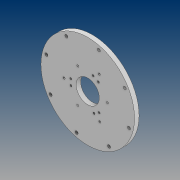
# Autodesk Inventor part: foreas_2_2_old
Saved by Autodesk Inventor 2021 (Build 250183000, 183)
## iProperties
Created: 2021-01-08
Part Number: foreas_2_2_old
Material: Generic
Document SubType Name: Modeling
Designer: Angelos
Density: 1 g/cm^3
Appearance: Default
Author: Angelos
Autodesk Inventor part; units mm, degrees
(part 1 of 3)
ref_plane "YZ Plane" through (0, 0, 0) normal (1, 0, 0) x (0, 1, 0)
ref_plane "XZ Plane" through (0, 0, 0) normal (0, 1, 0) x (-1, 0, 0)
ref_plane "XY Plane" through (0, 0, 0) normal (0, 0, 1) x (1, 0, 0)
sketch "Sketch2" plane through (0, 0, 0) normal (0, 0, 1) x (1, 0, 0)
  circle A0 centre (0, 0) radius 235
  circle A1 centre (115.1116, 204.8763) radius 10
  circle A2 centre (53.4628, 161.3745) radius 10
  circle A3 centre (0, 0) radius 170
  circle A4 centre (105.4319, 133.3571) radius 10
  circle A5 centre (115.1116, 204.8763) radius 10
  line L0 (114.1116, 214.8763) -> (115.1116, 213.4482)
  line L1 (115.1116, 213.4482) -> (116.1116, 214.8763)
  circle A6 centre (-234.9839, -2.7486) radius 10
  circle A7 centre (-166.4858, -34.3871) radius 10
  circle A8 centre (-168.2066, 24.6282) radius 10
  circle A9 centre (119.8723, -202.1278) radius 10
  circle A10 centre (113.023, -126.9874) radius 10
  circle A11 centre (62.7746, -157.9853) radius 10
  line L2 (107.6882, 200.5904) -> (105.9514, 200.7423)
  line L3 (106.9514, 199.0103) -> (107.6882, 200.5904)
  line L4 (122.5351, 200.5904) -> (123.2719, 199.0103)
  line L5 (124.2719, 200.7423) -> (122.5351, 200.5904)
  line L6 (-242.4074, -7.0345) -> (-244.1442, -6.8825)
  line L7 (-243.1442, -8.6146) -> (-242.4074, -7.0345)
  line L8 (-225.8237, -6.8825) -> (-227.5605, -7.0345)
  line L9 (-227.5605, -7.0345) -> (-226.8237, -8.6146)
  line L10 (-235.9839, 7.2514) -> (-234.9839, 5.8233)
  line L11 (-234.9839, 5.8233) -> (-233.9839, 7.2514)
  line L12 (127.2957, -206.4137) -> (128.0325, -207.9938)
  line L13 (129.0325, -206.2617) -> (127.2957, -206.4137)
  line L14 (118.8723, -192.1278) -> (119.8723, -193.5559)
  line L15 (119.8723, -193.5559) -> (120.8723, -192.1278)
  line L16 (111.712, -207.9938) -> (112.4488, -206.4137)
  line L17 (112.4488, -206.4137) -> (110.712, -206.2617)
  circle A12 centre (0, 0) radius 465
  circle A13 centre (0, 0) radius 196
  line L18 (0, 0) -> (105.4319, 133.3571)
  line L19 (119.8723, -202.1278) -> (0, 0)
  circle A14 centre (196, 0) radius 10
  line L20 (0, 0) -> (196, 0)
  circle A15 centre (-98, 169.741) radius 10
  circle A16 centre (-98, -169.741) radius 10
  point P0 (155.1924, 176.4662)
  point P1 (155.1924, 176.4662)
  point P2 (155.1924, 176.4662)
  point P3 (128.9755, -206.2667)
  point P4 (128.0083, -207.9419)
  point P5 (111.7362, -207.9419)
  point P6 (110.769, -206.2667)
  point P7 (118.9051, -192.1747)
  point P8 (120.8395, -192.1747)
  point P9 (123.2477, 199.0622)
  point P10 (106.9756, 199.0622)
  point P11 (106.0084, 200.7374)
  point P12 (114.1445, 214.8294)
  point P13 (116.0788, 214.8294)
  point P14 (124.2149, 200.7374)
  point P15 (-234.0168, 7.2046)
  point P16 (-225.8807, -6.8875)
  point P17 (-226.8479, -8.5627)
  point P18 (-243.12, -8.5627)
  point P19 (-244.0872, -6.8875)
  point P20 (-235.9511, 7.2046)
  dimension "d44" = 470
  dimension "d45" = 20
  dimension "d46" = 20
  dimension "d47" = 170
  dimension "d48" = 20
  dimension "d49" = 20
  dimension "d50" = 20
  dimension "d51" = 360
  dimension "d52" = 234.9839
  dimension "d55" = 360
  dimension "d59" = 360
  dimension "d61" = 930
  dimension "d76" = 392
  dimension "d84" = 20
  dimension "d94" = 360
  constraints: 42 end point, 16 centre point, 6 coincident, 2 point on circle, 91 other
  measures "d45" diameter of A1
  measures "d46" diameter of A2
  measures "d47" distance of A2.centre point (0, 0)
  measures "d48" diameter of A4
  measures "d50" diameter of A5
  measures "d52" horizontal distance of point (0, 0) A6.centre
  measures "d61" diameter of A12
  measures "d76" diameter of A13
  measures "d84" diameter of A14
extrude "Extrusion2" add sketch "Sketch2" along normal blind 20 contours A0 A9 A6 A1 | A1 L4 A0 | A0 L4 L5 A1 | L15 L14 A9 | A1 L2 L3 | L17 L16 A9 A0 | A0 A9 L17 | A9 L12 L13 | A6 L11 A0 | A0 L11 L10 A6 | A1 L1 L0 | L6 L7 A6 | L9 L8 A6 | A2 A3 A8 A7 A11 L19 A13 A16 A15 A14 L20 A4 | A2 A3 A4 L18 L19 A11 A7 A8 | A4 A3 L20 L18 | L20 A3 A10 L19 | L20 A14 A13 L19 A3 A10 | L20 A13 A14 | A14 A13 L20 | A14 A13 | A16 A13 | A13 A16 | A15 A13 | A13 A15 | A12
thread "Thread1" size "M20x2.5" class "6H" standard "ANSI Metric M Profile" full length
thread "Thread2" size "M20x2.5" class "6H" standard "ANSI Metric M Profile" full length
thread "Thread3" size "M20x2.5" class "6H" standard "ANSI Metric M Profile" full length
thread "Thread4" size "M20x2.5" class "6H" standard "ANSI Metric M Profile" full length
thread "Thread5" size "M20x2.5" class "6H" standard "ANSI Metric M Profile" full length
thread "Thread6" size "M20x2.5" class "6H" standard "ANSI Metric M Profile" full length
extrude "Extrusion3" cut sketch "Sketch2" along normal through all contours L20 A13 A14 | A14 A13 L20 | A14 A13 | A16 A13 | A13 A16 | A15 A13 | A13 A15
sketch "Sketch3" plane through (0, 0, 20) normal (0, 0, 1) x (1, 0, 0)
  circle A0 centre (0, 0) radius 115
  dimension "d96" = 230
  constraints: 1 centre point, 1 coincident
  measures "d96" diameter of A0
extrude "Extrusion4" cut sketch "Sketch3" against normal through all
sketch "Sketch4" plane through (0, 0, 20) normal (0, 0, 1) x (1, 0, 0)
  circle A0 centre (0, 0) radius 425
  circle A1 centre (110.6339, 410.3476) radius 15
  line L0 (0, 425) -> (110.6339, 410.3476)
  dimension "d103" = 360
  dimension "d99" = 850
  dimension "d112" = 111.6
  dimension "d113" = 0
  dimension "d114" = 0
  constraints: 3 point on circle, 2 centre point, 2 end point, 1 coincident, 1 other
  measures "d99" diameter of A0
  measures "d112" distance of L0.start L0.end
  measures "d113" distance of L0.end A1.centre
  measures "d114" horizontal distance of point (0, 0) L0.start
extrude "Extrusion5" cut sketch "Sketch4" against normal blind 50 contours A1 A0 | A0 L0 A1 | L0 A0 A1 picked at (104.0654, 411.4285) picked at (112.4556, 404.9089)
pattern_circular "Circular Pattern1" count 8 over 360 about axis through (0, 0, -10) along (0, 0, 1) of "Extrusion5"
sketch "Sketch6" plane through (0, 0, 0) normal (0, 0, -1) x (-1, 0, 0)
  circle A0 centre (0, 0) radius 465
  circle A1 centre (0, 0) radius 115
  dimension "d123" = 930
  constraints: 2 centre point, 2 coincident
  measures "d123" diameter of A0
extrude "Extrusion7" add sketch "Sketch6" along normal blind 25
sketch "Sketch7" plane through (0, 0, -25) normal (0, 0, -1) x (-1, 0, 0)
  circle A0 centre (0, 0) radius 130
  circle A1 centre (0, 130) radius 8
  circle A2 centre (-123.6373, 40.1722) radius 8
  circle A3 centre (-76.4121, -105.1722) radius 8
  circle A4 centre (76.4121, -105.1722) radius 8
  circle A5 centre (123.6373, 40.1722) radius 8
  dimension "d126" = 260
  dimension "d127" = 16
  dimension "d184" = 360
  constraints: 5 centre point, 1 coincident, 1 vertical alignment, 13 other
  measures "d127" diameter of A1
extrude "Extrusion8" cut sketch "Sketch7" against normal blind 15 contours A5 A0 | A0 A5 | A4 A0 | A0 A4 | A1 A0 | A0 A1 | A3 A0 | A0 A3 | A2 A0 | A0 A2
sketch "Sketch8" plane through (0, 0, 0) normal (1, 0, 0) x (0, 1, 0)
  line L0 (138, -10) -> (122, -10) projected
  line L1 (138, -10) -> (122, -10)
  line L2 (122, -10) -> (130, -2)
  line L3 (138, -10) -> (130, -2)
  line L4 (138, -10) -> (157.9972, -10) construction
  line L5 (138, -10) -> (130.4376, -10)
  line L6 (130, -2) -> (130, -10)
  line L7 (130, -2) -> (138, -2) construction
  point P0 (0, 0)
  dimension "d176" = 45
  dimension "d177" = 135
  dimension "d178" = 90
  constraints: 14 end point, 2 collinear, 2 horizontal, 1 midpoint, 1 perpendicular, 1 point on line
  measures "d176" angle of L1 L2
  measures "d177" angle of L4 L3
  measures "d178" angle of L6 L7
revolve "Revolution1" cut sketch "Sketch8" angle 360 about axis through (0, 130, -2) along (0, 0, -1) contours L0 L6 L3
pattern_circular "Circular Pattern3" count 5 over 360 about axis through (0, 0, 20) along (0, 0, -1) of "Revolution1"
sketch "Sketch9" plane through (0, 0, 20) normal (0, 0, 1) x (1, 0, 0)
  circle A0 centre (-166.4858, -34.3871) radius 10 projected
  circle A1 centre (-166.4858, -34.3871) radius 10
  circle A2 centre (-168.2066, 24.6282) radius 10 projected
  circle A3 centre (-168.2066, 24.6282) radius 10
  point P0 (0, 0)
  constraints: 2 centre point, 2 coincident
extrude "Extrusion9" cut sketch "Sketch9" against normal through all
pattern_circular "Circular Pattern4" count 3 over 360 about axis through (0, 0, 20) along (0, 0, -1) of "Extrusion9"
sketch "Sketch10" plane through (0, 0, 20) normal (0, 0, 1) x (1, 0, 0)
  circle A0 centre (-368.3896, -211.9296) radius 15 projected
  circle A1 centre (-368.3896, -211.9296) radius 15
  point P0 (0, 0)
  constraints: 1 centre point, 1 coincident
extrude "Extrusion10" cut sketch "Sketch10" against normal through all
pattern_circular "Circular Pattern5" count 8 over 360 about axis through (0, 0, 20) along (0, 0, -1) of "Extrusion10"
thread "Thread7" size "M30x3.5" class "6H" standard "ANSI Metric M Profile" full length
thread "Thread8" size "M30x3.5" class "6H" standard "ANSI Metric M Profile" full length
thread "Thread9" size "M30x3.5" class "6H" standard "ANSI Metric M Profile" full length
thread "Thread10" size "M30x3.5" class "6H" standard "ANSI Metric M Profile" full length
thread "Thread11" size "M30x3.5" class "6H" standard "ANSI Metric M Profile" full length
thread "Thread12" size "M30x3.5" class "6H" standard "ANSI Metric M Profile" full length
thread "Thread13" size "M30x3.5" class "6H" standard "ANSI Metric M Profile" full length
thread "Thread14" size "M30x3.5" class "6H" standard "ANSI Metric M Profile" full length
thread "Thread15" size "M20x2.5" class "6H" standard "ANSI Metric M Profile" full length
thread "Thread16" size "M20x2.5" class "6H" standard "ANSI Metric M Profile" full length
thread "Thread17" size "M20x2.5" class "6H" standard "ANSI Metric M Profile" full length
thread "Thread18" size "M20x2.5" class "6H" standard "ANSI Metric M Profile" full length
thread "Thread19" size "M20x2.5" class "6H" standard "ANSI Metric M Profile" full length
thread "Thread20" size "M20x2.5" class "6H" standard "ANSI Metric M Profile" full length
pattern_circular "Circular Pattern6" count 5 over 360 about axis through (0, 0, -10) along (0, 0, 1) of "Revolution1"
thread "Thread21" size "M16x2" class "6H" standard "ANSI Metric M Profile" full length
thread "Thread22" size "M16x2" class "6H" standard "ANSI Metric M Profile" full length
thread "Thread23" size "M16x2" class "6H" standard "ANSI Metric M Profile" full length
thread "Thread24" size "M16x2" class "6H" standard "ANSI Metric M Profile" full length
thread "Thread25" size "M16x2" class "6H" standard "ANSI Metric M Profile" full length
sketch "Sketch11" plane through (0, 0, -25) normal (0, 0, -1) x (-1, 0, 0)
  circle A0 centre (0, 0) radius 115 projected
  circle A1 centre (0, 0) radius 318.114
  circle A2 centre (0, 0) radius 359.1006
  spline S0 degree 2 poles (-321.1231, 5.4547) (-320.2877, 5.4473) (-318.9493, 4.758) (-318.5787, 4.1862) knots 0 0 0 1 2 2 2
  spline S1 degree 2 poles (-318.5787, 4.1862) (-318.2912, 3.719) (-318.102, 2.7632) (-318.1087, 2.0217) knots 0 0 0 1 2 2 2
  line L0 (-318.1087, 2.0217) -> (-318.1212, 0.6179)
  line L1 (-318.1212, 0.6179) -> (-324.221, 0.6724)
  line L2 (-324.221, 0.6724) -> (-324.2085, 2.0614)
  spline S2 degree 2 poles (-324.2085, 2.0614) (-324.2008, 2.9215) (-323.9351, 3.898) (-323.7046, 4.2419) knots 0 0 0 1 2 2 2
  spline S3 degree 2 poles (-323.7046, 4.2419) (-323.3088, 4.8267) (-322.0129, 5.4627) (-321.1231, 5.4547) knots 0 0 0 1 2 2 2
  spline S4 degree 2 poles (-321.1406, 4.6096) (-321.8425, 4.6158) (-322.8402, 4.1601) (-323.1261, 3.7029) knots 0 0 0 1 2 2 2
  spline S5 degree 2 poles (-323.1261, 3.7029) (-323.3218, 3.3784) (-323.5014, 2.6434) (-323.5063, 2.0947) knots 0 0 0 1 2 2 2
  line L3 (-323.5063, 2.0947) -> (-323.5118, 1.4768)
  line L4 (-323.5118, 1.4768) -> (-318.8159, 1.4348)
  line L5 (-318.8159, 1.4348) -> (-318.8103, 2.0527)
  spline S6 degree 2 poles (-318.8103, 2.0527) (-318.8055, 2.5915) (-318.9712, 3.4087) (-319.2006, 3.7419) knots 0 0 0 1 2 2 2
  spline S7 degree 2 poles (-319.2006, 3.7419) (-319.4835, 4.1696) (-320.4288, 4.6032) (-321.1406, 4.6096) knots 0 0 0 1 2 2 2
  line L6 (-318.0044, 8.4321) -> (-318.0583, 6.0699)
  line L7 (-318.0583, 6.0699) -> (-318.681, 6.0841)
  line L8 (-318.681, 6.0841) -> (-318.6633, 6.8599)
  line L9 (-318.6633, 6.8599) -> (-323.5163, 6.9706)
  line L10 (-323.5163, 6.9706) -> (-323.534, 6.1947)
  line L11 (-323.534, 6.1947) -> (-324.1567, 6.2089)
  line L12 (-324.1567, 6.2089) -> (-324.1028, 8.5712)
  line L13 (-324.1028, 8.5712) -> (-323.4801, 8.557)
  line L14 (-323.4801, 8.557) -> (-323.4978, 7.7811)
  line L15 (-323.4978, 7.7811) -> (-318.6448, 7.6704)
  line L16 (-318.6448, 7.6704) -> (-318.6271, 8.4463)
  line L17 (-318.6271, 8.4463) -> (-318.0044, 8.4321)
  spline S8 degree 2 poles (-323.2222, 13.948) (-322.8043, 14.2788) (-321.6044, 14.6202) (-320.8437, 14.592) knots 0 0 0 1 2 2 2
  spline S9 degree 2 poles (-320.8437, 14.592) (-320.1027, 14.5645) (-318.9162, 14.1446) (-318.5243, 13.7739) knots 0 0 0 1 2 2 2
  spline S10 degree 2 poles (-318.5243, 13.7739) (-318.1134, 13.3827) (-317.7452, 12.3748) (-317.7673, 11.777) knots 0 0 0 1 2 2 2
  spline S11 degree 2 poles (-317.7673, 11.777) (-317.7902, 11.1596) (-318.2467, 10.1871) (-318.6701, 9.8417) knots 0 0 0 1 2 2 2
  spline S12 degree 2 poles (-318.6701, 9.8417) (-319.0882, 9.506) (-320.2926, 9.1747) (-321.0435, 9.2026) knots 0 0 0 1 2 2 2
  spline S13 degree 2 poles (-321.0435, 9.2026) (-321.8091, 9.2309) (-322.9609, 9.6545) (-323.3677, 10.0208) knots 0 0 0 1 2 2 2
  spline S14 degree 2 poles (-323.3677, 10.0208) (-323.7596, 10.3915) (-324.1427, 11.4) (-324.12, 12.0125) knots 0 0 0 1 2 2 2
  spline S15 degree 2 poles (-324.12, 12.0125) (-324.0969, 12.635) (-323.6252, 13.6167) (-323.2222, 13.948) knots 0 0 0 1 2 2 2
  spline S16 degree 2 poles (-320.875, 13.7472) (-321.4777, 13.7696) (-322.421, 13.5424) (-322.7361, 13.3166) knots 0 0 0 1 2 2 2
  spline S17 degree 2 poles (-322.7361, 13.3166) (-323.0612, 13.0863) (-323.4026, 12.4163) (-323.4184, 11.9915) knots 0 0 0 1 2 2 2
  spline S18 degree 2 poles (-323.4184, 11.9915) (-323.4347, 11.5518) (-323.1529, 10.8785) (-322.8362, 10.6145) knots 0 0 0 1 2 2 2
  spline S19 degree 2 poles (-322.8362, 10.6145) (-322.534, 10.3609) (-321.6049, 10.0693) (-321.0122, 10.0473) knots 0 0 0 1 2 2 2
  spline S20 degree 2 poles (-321.0122, 10.0473) (-319.8118, 10.0028) (-318.4999, 10.9633) (-318.4686, 11.808) knots 0 0 0 1 2 2 2
  spline S21 degree 2 poles (-318.4686, 11.808) (-318.4373, 12.6527) (-319.6746, 13.7027) (-320.875, 13.7472) knots 0 0 0 1 2 2 2
  spline S22 degree 2 poles (-317.4907, 17.9128) (-317.5264, 17.2662) (-317.9804, 16.217) (-318.4015, 15.8541) knots 0 0 0 1 2 2 2
  spline S23 degree 2 poles (-318.4015, 15.8541) (-318.8275, 15.4915) (-320.0446, 15.1478) (-320.8195, 15.1906) knots 0 0 0 1 2 2 2
  spline S24 degree 2 poles (-320.8195, 15.1906) (-321.5549, 15.2312) (-322.6968, 15.7102) (-323.0902, 16.118) knots 0 0 0 1 2 2 2
  spline S25 degree 2 poles (-323.0902, 16.118) (-323.4695, 16.5103) (-323.8439, 17.6202) (-323.8082, 18.2668) knots 0 0 0 1 2 2 2
  spline S26 degree 2 poles (-323.8082, 18.2668) (-323.791, 18.5777) (-323.6711, 19.1355) (-323.5779, 19.3878) knots 0 0 0 1 2 2 2
  spline S27 degree 2 poles (-323.5779, 19.3878) (-323.5072, 19.5918) (-323.2622, 20.0833) (-323.1748, 20.2319) knots 0 0 0 1 2 2 2
  line L18 (-323.1748, 20.2319) -> (-322.1975, 20.1779)
  line L19 (-322.1975, 20.1779) -> (-322.2014, 20.1088)
  spline S28 degree 2 poles (-322.2014, 20.1088) (-322.3431, 19.9632) (-322.6026, 19.6557) (-322.7572, 19.3672) knots 0 0 0 1 2 2 2
  spline S29 degree 2 poles (-322.7572, 19.3672) (-322.8942, 19.1272) (-323.0923, 18.4995) (-323.1125, 18.1343) knots 0 0 0 1 2 2 2
  spline S30 degree 2 poles (-323.1125, 18.1343) (-323.161, 17.2557) (-321.8982, 16.0968) (-320.7975, 16.036) knots 0 0 0 1 2 2 2
  spline S31 degree 2 poles (-320.7975, 16.036) (-320.1855, 16.0021) (-319.2516, 16.2377) (-318.9207, 16.4917) knots 0 0 0 1 2 2 2
  spline S32 degree 2 poles (-318.9207, 16.4917) (-318.5904, 16.7359) (-318.2188, 17.458) (-318.1932, 17.9219) knots 0 0 0 1 2 2 2
  spline S33 degree 2 poles (-318.1932, 17.9219) (-318.1744, 18.2625) (-318.2355, 18.9491) (-318.3214, 19.1865) knots 0 0 0 1 2 2 2
  line L20 (-318.3214, 19.1865) -> (-319.8959, 19.2735)
  line L21 (-319.8959, 19.2735) -> (-319.9738, 17.8619)
  line L22 (-319.9738, 17.8619) -> (-320.6846, 17.9011)
  line L23 (-320.6846, 17.9011) -> (-320.5624, 20.1123)
  line L24 (-320.5624, 20.1123) -> (-317.9021, 19.9654)
  spline S34 degree 2 poles (-317.9021, 19.9654) (-317.8414, 19.8085) (-317.6581, 19.2736) (-317.6062, 19.048) knots 0 0 0 1 2 2 2
  spline S35 degree 2 poles (-317.6062, 19.048) (-317.534, 18.742) (-317.4719, 18.2534) (-317.4907, 17.9128) knots 0 0 0 1 2 2 2
  line L25 (-317.4276, 20.9589) -> (-323.512, 21.394)
  line L26 (-323.512, 21.394) -> (-323.2398, 25.2005)
  line L27 (-323.2398, 25.2005) -> (-322.52, 25.149)
  line L28 (-322.52, 25.149) -> (-322.7343, 22.1512)
  line L29 (-322.7343, 22.1512) -> (-321.0678, 22.032)
  line L30 (-321.0678, 22.032) -> (-320.8678, 24.8277)
  line L31 (-320.8678, 24.8277) -> (-320.148, 24.7762)
  line L32 (-320.148, 24.7762) -> (-320.3479, 21.9805)
  line L33 (-320.3479, 21.9805) -> (-318.0896, 21.819)
  line L34 (-318.0896, 21.819) -> (-317.8753, 24.8169)
  line L35 (-317.8753, 24.8169) -> (-317.1554, 24.7654)
  line L36 (-317.1554, 24.7654) -> (-317.4276, 20.9589)
  line L37 (-316.7037, 30.0006) -> (-316.7833, 29.0945)
  line L38 (-316.7833, 29.0945) -> (-322.2589, 26.8659)
  line L39 (-322.2589, 26.8659) -> (-317.0194, 26.4058)
  line L40 (-317.0194, 26.4058) -> (-317.0855, 25.6524)
  line L41 (-317.0855, 25.6524) -> (-323.1622, 26.186)
  line L42 (-323.1622, 26.186) -> (-323.0614, 27.3334)
  line L43 (-323.0614, 27.3334) -> (-318.0354, 29.3583)
  line L44 (-318.0354, 29.3583) -> (-322.8465, 29.7808)
  line L45 (-322.8465, 29.7808) -> (-322.7803, 30.5342)
  line L46 (-322.7803, 30.5342) -> (-316.7037, 30.0006)
  line L47 (-316.3638, 33.3448) -> (-316.6027, 30.994)
  line L48 (-316.6027, 30.994) -> (-317.2224, 31.057)
  line L49 (-317.2224, 31.057) -> (-317.1439, 31.8291)
  line L50 (-317.1439, 31.8291) -> (-321.9733, 32.32)
  line L51 (-321.9733, 32.32) -> (-322.0518, 31.5479)
  line L52 (-322.0518, 31.5479) -> (-322.6715, 31.6109)
  line L53 (-322.6715, 31.6109) -> (-322.4325, 33.9617)
  line L54 (-322.4325, 33.9617) -> (-321.8128, 33.8987)
  line L55 (-321.8128, 33.8987) -> (-321.8913, 33.1266)
  line L56 (-321.8913, 33.1266) -> (-317.0619, 32.6356)
  line L57 (-317.0619, 32.6356) -> (-316.9834, 33.4078)
  line L58 (-316.9834, 33.4078) -> (-316.3638, 33.3448)
  spline S36 degree 2 poles (-315.9587, 36.02) (-316.0338, 35.3619) (-316.4141, 34.4699) (-316.6571, 34.0847) knots 0 0 0 1 2 2 2
  line L59 (-316.6571, 34.0847) -> (-317.6688, 34.2001)
  line L60 (-317.6688, 34.2001) -> (-317.6621, 34.259)
  spline S37 degree 2 poles (-317.6621, 34.259) (-317.2435, 34.6142) (-316.7161, 35.574) (-316.6629, 36.0406) knots 0 0 0 1 2 2 2
  spline S38 degree 2 poles (-316.6629, 36.0406) (-316.5867, 36.7086) (-317.0638, 37.4546) (-317.5206, 37.5067) knots 0 0 0 1 2 2 2
  spline S39 degree 2 poles (-317.5206, 37.5067) (-317.884, 37.5481) (-318.3767, 37.2411) (-318.534, 36.866) knots 0 0 0 1 2 2 2
  spline S40 degree 2 poles (-318.534, 36.866) (-318.6445, 36.595) (-318.8057, 36.1407) (-318.9339, 35.8021) knots 0 0 0 1 2 2 2
  spline S41 degree 2 poles (-318.9339, 35.8021) (-319.0533, 35.4973) (-319.3603, 35.0298) (-319.5835, 34.8612) knots 0 0 0 1 2 2 2
  spline S42 degree 2 poles (-319.5835, 34.8612) (-319.8062, 34.6976) (-320.37, 34.5529) (-320.7236, 34.5932) knots 0 0 0 1 2 2 2
  spline S43 degree 2 poles (-320.7236, 34.5932) (-321.4603, 34.6773) (-322.3263, 35.9403) (-322.2249, 36.8292) knots 0 0 0 1 2 2 2
  spline S44 degree 2 poles (-322.2249, 36.8292) (-322.1666, 37.34) (-321.8622, 38.2208) (-321.6264, 38.5869) knots 0 0 0 1 2 2 2
  line L61 (-321.6264, 38.5869) -> (-320.6637, 38.4771)
  line L62 (-320.6637, 38.4771) -> (-320.6705, 38.4182)
  spline S45 degree 2 poles (-320.6705, 38.4182) (-320.9687, 38.1587) (-321.4647, 37.2998) (-321.5213, 36.8037) knots 0 0 0 1 2 2 2
  spline S46 degree 2 poles (-321.5213, 36.8037) (-321.5851, 36.2438) (-321.1386, 35.4914) (-320.7113, 35.4426) knots 0 0 0 1 2 2 2
  spline S47 degree 2 poles (-320.7113, 35.4426) (-320.3282, 35.3989) (-319.825, 35.7545) (-319.6781, 36.1258) knots 0 0 0 1 2 2 2
  spline S48 degree 2 poles (-319.6781, 36.1258) (-319.5802, 36.3734) (-319.3188, 37.0948) (-319.2172, 37.332) knots 0 0 0 1 2 2 2
  spline S49 degree 2 poles (-319.2172, 37.332) (-318.9545, 37.9339) (-318.1173, 38.4255) (-317.5525, 38.3611) knots 0 0 0 1 2 2 2
  spline S50 degree 2 poles (-317.5525, 38.3611) (-317.1939, 38.3202) (-316.5394, 37.952) (-316.3284, 37.6642) knots 0 0 0 1 2 2 2
  spline S51 degree 2 poles (-316.3284, 37.6642) (-316.0962, 37.3442) (-315.8954, 36.575) (-315.9587, 36.02) knots 0 0 0 1 2 2 2
  line L63 (-315.1957, 42.9923) -> (-320.5237, 43.726)
  line L64 (-320.5237, 43.726) -> (-320.8029, 41.6987)
  line L65 (-320.8029, 41.6987) -> (-321.5179, 41.7971)
  line L66 (-321.5179, 41.7971) -> (-320.8489, 46.655)
  line L67 (-320.8489, 46.655) -> (-320.1339, 46.5565)
  line L68 (-320.1339, 46.5565) -> (-320.4131, 44.5292)
  line L69 (-320.4131, 44.5292) -> (-315.0851, 43.7954)
  line L70 (-315.0851, 43.7954) -> (-315.1957, 42.9923)
  spline S52 degree 2 poles (-314.3461, 48.1028) (-314.4463, 47.448) (-314.8606, 46.5713) (-315.1181, 46.1956) knots 0 0 0 1 2 2 2
  line L71 (-315.1181, 46.1956) -> (-316.1247, 46.3497)
  line L72 (-316.1247, 46.3497) -> (-316.1157, 46.4084)
  spline S53 degree 2 poles (-316.1157, 46.4084) (-315.6838, 46.7473) (-315.12, 47.6862) (-315.0489, 48.1504) knots 0 0 0 1 2 2 2
  spline S54 degree 2 poles (-315.0489, 48.1504) (-314.9472, 48.8149) (-315.3954, 49.5787) (-315.8498, 49.6482) knots 0 0 0 1 2 2 2
  spline S55 degree 2 poles (-315.8498, 49.6482) (-316.2114, 49.7036) (-316.7156, 49.4157) (-316.887, 49.0469) knots 0 0 0 1 2 2 2
  spline S56 degree 2 poles (-316.887, 49.0469) (-317.0079, 48.7803) (-317.1864, 48.3326) (-317.3275, 47.9991) knots 0 0 0 1 2 2 2
  spline S57 degree 2 poles (-317.3275, 47.9991) (-317.4584, 47.6991) (-317.7832, 47.2437) (-318.0127, 47.0838) knots 0 0 0 1 2 2 2
  spline S58 degree 2 poles (-318.0127, 47.0838) (-318.2414, 46.9288) (-318.8104, 46.8059) (-319.1622, 46.8597) knots 0 0 0 1 2 2 2
  spline S59 degree 2 poles (-319.1622, 46.8597) (-319.8951, 46.9719) (-320.712, 48.2672) (-320.5766, 49.1516) knots 0 0 0 1 2 2 2
  spline S60 degree 2 poles (-320.5766, 49.1516) (-320.4988, 49.6598) (-320.1609, 50.5282) (-319.9112, 50.8851) knots 0 0 0 1 2 2 2
  line L73 (-319.9112, 50.8851) -> (-318.9535, 50.7384)
  line L74 (-318.9535, 50.7384) -> (-318.9625, 50.6798)
  spline S61 degree 2 poles (-318.9625, 50.6798) (-319.2705, 50.4319) (-319.799, 49.5927) (-319.8745, 49.0991) knots 0 0 0 1 2 2 2
  spline S62 degree 2 poles (-319.8745, 49.0991) (-319.9598, 48.5421) (-319.5424, 47.7731) (-319.1173, 47.708) knots 0 0 0 1 2 2 2
  spline S63 degree 2 poles (-319.1173, 47.708) (-318.7362, 47.6497) (-318.2197, 47.9857) (-318.0587, 48.3511) knots 0 0 0 1 2 2 2
  spline S64 degree 2 poles (-318.0587, 48.3511) (-317.9514, 48.5947) (-317.6626, 49.3056) (-317.5519, 49.5387) knots 0 0 0 1 2 2 2
  spline S65 degree 2 poles (-317.5519, 49.5387) (-317.2663, 50.1301) (-316.4109, 50.5893) (-315.849, 50.5032) knots 0 0 0 1 2 2 2
  spline S66 degree 2 poles (-315.849, 50.5032) (-315.4922, 50.4486) (-314.8523, 50.0556) (-314.6525, 49.76) knots 0 0 0 1 2 2 2
  spline S67 degree 2 poles (-314.6525, 49.76) (-314.4328, 49.4313) (-314.2616, 48.655) (-314.3461, 48.1028) knots 0 0 0 1 2 2 2
  line L75 (-313.6445, 53.1511) -> (-314.0307, 50.8199)
  line L76 (-314.0307, 50.8199) -> (-314.6451, 50.9217)
  line L77 (-314.6451, 50.9217) -> (-314.5183, 51.6874)
  line L78 (-314.5183, 51.6874) -> (-319.3073, 52.4807)
  line L79 (-319.3073, 52.4807) -> (-319.4342, 51.715)
  line L80 (-319.4342, 51.715) -> (-320.0487, 51.8168)
  line L81 (-320.0487, 51.8168) -> (-319.6625, 54.148)
  line L82 (-319.6625, 54.148) -> (-319.048, 54.0462)
  line L83 (-319.048, 54.0462) -> (-319.1749, 53.2805)
  line L84 (-319.1749, 53.2805) -> (-314.3858, 52.4872)
  line L85 (-314.3858, 52.4872) -> (-314.259, 53.2528)
  line L86 (-314.259, 53.2528) -> (-313.6445, 53.1511)
  spline S68 degree 2 poles (-312.9522, 56.467) (-313.0566, 55.8831) (-313.6274, 54.9658) (-314.086, 54.6762) knots 0 0 0 1 2 2 2
  spline S69 degree 2 poles (-314.086, 54.6762) (-314.5397, 54.3857) (-315.778, 54.2005) (-316.5371, 54.3363) knots 0 0 0 1 2 2 2
  spline S70 degree 2 poles (-316.5371, 54.3363) (-317.2914, 54.4712) (-318.3418, 55.0558) (-318.6901, 55.4947) knots 0 0 0 1 2 2 2
  spline S71 degree 2 poles (-318.6901, 55.4947) (-319.0296, 55.927) (-319.2771, 56.9857) (-319.1684, 57.594) knots 0 0 0 1 2 2 2
  spline S72 degree 2 poles (-319.1684, 57.594) (-319.1144, 57.8957) (-318.9319, 58.4104) (-318.8238, 58.622) knots 0 0 0 1 2 2 2
  spline S73 degree 2 poles (-318.8238, 58.622) (-318.7257, 58.8054) (-318.4734, 59.1771) (-318.3307, 59.3574) knots 0 0 0 1 2 2 2
  line L87 (-318.3307, 59.3574) -> (-317.3672, 59.1851)
  line L88 (-317.3672, 59.1851) -> (-317.3785, 59.1218)
  spline S74 degree 2 poles (-317.3785, 59.1218) (-317.495, 59.0322) (-317.8267, 58.75) (-318.0007, 58.5351) knots 0 0 0 1 2 2 2
  spline S75 degree 2 poles (-318.0007, 58.5351) (-318.1681, 58.329) (-318.4253, 57.8176) (-318.488, 57.4672) knots 0 0 0 1 2 2 2
  spline S76 degree 2 poles (-318.488, 57.4672) (-318.5567, 57.0828) (-318.3632, 56.3401) (-318.1076, 56.0283) knots 0 0 0 1 2 2 2
  spline S77 degree 2 poles (-318.1076, 56.0283) (-317.8463, 55.7204) (-316.9674, 55.2719) (-316.3883, 55.1684) knots 0 0 0 1 2 2 2
  spline S78 degree 2 poles (-316.3883, 55.1684) (-315.7703, 55.0578) (-314.8267, 55.1954) (-314.4741, 55.3984) knots 0 0 0 1 2 2 2
  spline S79 degree 2 poles (-314.4741, 55.3984) (-314.132, 55.5984) (-313.7093, 56.2208) (-313.6414, 56.6003) knots 0 0 0 1 2 2 2
  spline S80 degree 2 poles (-313.6414, 56.6003) (-313.5796, 56.9458) (-313.6446, 57.5651) (-313.7302, 57.8164) knots 0 0 0 1 2 2 2
  spline S81 degree 2 poles (-313.7302, 57.8164) (-313.8176, 58.058) (-314.022, 58.4311) (-314.0979, 58.54) knots 0 0 0 1 2 2 2
  line L89 (-314.0979, 58.54) -> (-314.0875, 58.5984)
  line L90 (-314.0875, 58.5984) -> (-313.1337, 58.4278)
  spline S82 degree 2 poles (-313.1337, 58.4278) (-313.077, 58.2118) (-312.9693, 57.831) (-312.9359, 57.5689) knots 0 0 0 1 2 2 2
  spline S83 degree 2 poles (-312.9359, 57.5689) (-312.8953, 57.2904) (-312.8877, 56.8271) (-312.9522, 56.467) knots 0 0 0 1 2 2 2
  line L91 (-311.7311, 63.444) -> (-311.8873, 62.6485)
  line L92 (-311.8873, 62.6485) -> (-314.8171, 63.2236)
  line L93 (-314.8171, 63.2236) -> (-315.3579, 60.4684)
  line L94 (-315.3579, 60.4684) -> (-312.428, 59.8933)
  line L95 (-312.428, 59.8933) -> (-312.5842, 59.0978)
  line L96 (-312.5842, 59.0978) -> (-318.57, 60.2727)
  line L97 (-318.57, 60.2727) -> (-318.4138, 61.0682)
  line L98 (-318.4138, 61.0682) -> (-316.0661, 60.6074)
  line L99 (-316.0661, 60.6074) -> (-315.5253, 63.3626)
  line L100 (-315.5253, 63.3626) -> (-317.873, 63.8234)
  line L101 (-317.873, 63.8234) -> (-317.7169, 64.6189)
  line L102 (-317.7169, 64.6189) -> (-311.7311, 63.444)
  line L103 (-310.7438, 68.111) -> (-311.4781, 64.6536)
  line L104 (-311.4781, 64.6536) -> (-317.445, 65.921)
  line L105 (-317.445, 65.921) -> (-317.2765, 66.714)
  line L106 (-317.2765, 66.714) -> (-312.0156, 65.5966)
  line L107 (-312.0156, 65.5966) -> (-311.4497, 68.2609)
  line L108 (-311.4497, 68.2609) -> (-310.7438, 68.111)
  line L109 (-310.7518, 68.0925) -> (-316.243, 71.4518)
  line L110 (-316.243, 71.4518) -> (-316.0213, 72.4254)
  line L111 (-316.0213, 72.4254) -> (-309.617, 73.0763)
  line L112 (-309.617, 73.0763) -> (-309.8069, 72.2424)
  line L113 (-309.8069, 72.2424) -> (-311.5927, 72.0812)
  line L114 (-311.5927, 72.0812) -> (-312.1096, 69.811)
  line L115 (-312.1096, 69.811) -> (-310.5696, 68.8926)
  line L116 (-310.5696, 68.8926) -> (-310.7518, 68.0925)
  line L117 (-312.3169, 72.018) -> (-315.3268, 71.735)
  line L118 (-315.3268, 71.735) -> (-312.735, 70.1816)
  line L119 (-312.735, 70.1816) -> (-312.3169, 72.018)
  line L120 (-308.4049, 78.0367) -> (-308.6548, 77.0139)
  line L121 (-308.6548, 77.0139) -> (-311.9403, 75.5217)
  line L122 (-311.9403, 75.5217) -> (-311.6359, 75.0809)
  line L123 (-311.6359, 75.0809) -> (-309.2685, 74.5025)
  line L124 (-309.2685, 74.5025) -> (-309.4609, 73.7149)
  line L125 (-309.4609, 73.7149) -> (-315.3866, 75.1629)
  line L126 (-315.3866, 75.1629) -> (-315.1941, 75.9504)
  line L127 (-315.1941, 75.9504) -> (-312.4714, 75.2851)
  line L128 (-312.4714, 75.2851) -> (-314.6004, 78.3802)
  line L129 (-314.6004, 78.3802) -> (-314.3657, 79.3406)
  line L130 (-314.3657, 79.3406) -> (-312.3194, 76.2403)
  line L131 (-312.3194, 76.2403) -> (-308.4049, 78.0367)
  line L132 (-307.746, 80.5623) -> (-308.336, 78.2742)
  line L133 (-308.336, 78.2742) -> (-308.9391, 78.4297)
  line L134 (-308.9391, 78.4297) -> (-308.7453, 79.1813)
  line L135 (-308.7453, 79.1813) -> (-313.4459, 80.3932)
  line L136 (-313.4459, 80.3932) -> (-313.6397, 79.6417)
  line L137 (-313.6397, 79.6417) -> (-314.2428, 79.7972)
  line L138 (-314.2428, 79.7972) -> (-313.6529, 82.0852)
  line L139 (-313.6529, 82.0852) -> (-313.0498, 81.9297)
  line L140 (-313.0498, 81.9297) -> (-313.2435, 81.1782)
  line L141 (-313.2435, 81.1782) -> (-308.5429, 79.9663)
  line L142 (-308.5429, 79.9663) -> (-308.3492, 80.7178)
  line L143 (-308.3492, 80.7178) -> (-307.746, 80.5623)
  spline S84 degree 2 poles (-306.9431, 83.1461) (-307.1163, 82.5068) (-307.6265, 81.6822) (-307.9247, 81.3379) knots 0 0 0 1 2 2 2
  line L144 (-307.9247, 81.3379) -> (-308.9076, 81.6042)
  line L145 (-308.9076, 81.6042) -> (-308.8921, 81.6615)
  spline S85 degree 2 poles (-308.8921, 81.6615) (-308.4247, 81.9497) (-307.7589, 82.8192) (-307.6361, 83.2725) knots 0 0 0 1 2 2 2
  spline S86 degree 2 poles (-307.6361, 83.2725) (-307.4603, 83.9214) (-307.8198, 84.7306) (-308.2635, 84.8509) knots 0 0 0 1 2 2 2
  spline S87 degree 2 poles (-308.2635, 84.8509) (-308.6166, 84.9465) (-309.1499, 84.7172) (-309.3618, 84.37) knots 0 0 0 1 2 2 2
  spline S88 degree 2 poles (-309.3618, 84.37) (-309.5118, 84.1187) (-309.7396, 83.6938) (-309.9172, 83.3784) knots 0 0 0 1 2 2 2
  spline S89 degree 2 poles (-309.9172, 83.3784) (-310.0811, 83.095) (-310.455, 82.679) (-310.701, 82.5459) knots 0 0 0 1 2 2 2
  spline S90 degree 2 poles (-310.701, 82.5459) (-310.9458, 82.4176) (-311.5249, 82.3594) (-311.8684, 82.4525) knots 0 0 0 1 2 2 2
  spline S91 degree 2 poles (-311.8684, 82.4525) (-312.5841, 82.6464) (-313.2502, 84.0253) (-313.0162, 84.8889) knots 0 0 0 1 2 2 2
  spline S92 degree 2 poles (-313.0162, 84.8889) (-312.8817, 85.3851) (-312.4483, 86.21) (-312.1601, 86.5365) knots 0 0 0 1 2 2 2
  line L146 (-312.1601, 86.5365) -> (-311.2249, 86.2832)
  line L147 (-311.2249, 86.2832) -> (-311.2404, 86.2259)
  spline S93 degree 2 poles (-311.2404, 86.2259) (-311.5743, 86.0142) (-312.1939, 85.2397) (-312.3244, 84.7578) knots 0 0 0 1 2 2 2
  spline S94 degree 2 poles (-312.3244, 84.7578) (-312.4718, 84.2139) (-312.1436, 83.4028) (-311.7285, 83.2904) knots 0 0 0 1 2 2 2
  spline S95 degree 2 poles (-311.7285, 83.2904) (-311.3563, 83.1895) (-310.8053, 83.4653) (-310.6043, 83.8103) knots 0 0 0 1 2 2 2
  spline S96 degree 2 poles (-310.6043, 83.8103) (-310.4702, 84.0403) (-310.1033, 84.7143) (-309.9671, 84.9334) knots 0 0 0 1 2 2 2
  spline S97 degree 2 poles (-309.9671, 84.9334) (-309.6168, 85.489) (-308.7152, 85.849) (-308.1665, 85.7004) knots 0 0 0 1 2 2 2
  spline S98 degree 2 poles (-308.1665, 85.7004) (-307.8182, 85.606) (-307.2265, 85.1435) (-307.0612, 84.8273) knots 0 0 0 1 2 2 2
  spline S99 degree 2 poles (-307.0612, 84.8273) (-306.8798, 84.476) (-306.797, 83.6853) (-306.9431, 83.1461) knots 0 0 0 1 2 2 2
  spline S100 degree 2 poles (-306.3956, 92.6511) (-305.9453, 92.518) (-305.2703, 91.9938) (-305.0886, 91.6669) knots 0 0 0 1 2 2 2
  spline S101 degree 2 poles (-305.0886, 91.6669) (-304.8954, 91.3263) (-304.8091, 90.5894) (-304.9253, 90.196) knots 0 0 0 1 2 2 2
  spline S102 degree 2 poles (-304.9253, 90.196) (-305.0416, 89.8025) (-305.499, 89.2315) (-305.8374, 89.0634) knots 0 0 0 1 2 2 2
  spline S103 degree 2 poles (-305.8374, 89.0634) (-306.2447, 88.8539) (-307.4122, 88.8278) (-308.1896, 89.0576) knots 0 0 0 1 2 2 2
  spline S104 degree 2 poles (-308.1896, 89.0576) (-308.9528, 89.2832) (-310.0882, 89.9589) (-310.4466, 90.4205) knots 0 0 0 1 2 2 2
  spline S105 degree 2 poles (-310.4466, 90.4205) (-310.7983, 90.8698) (-310.9991, 92.0219) (-310.8043, 92.6809) knots 0 0 0 1 2 2 2
  spline S106 degree 2 poles (-310.8043, 92.6809) (-310.7469, 92.8752) (-310.6081, 93.2054) (-310.5276, 93.3207) knots 0 0 0 1 2 2 2
  line L148 (-310.5276, 93.3207) -> (-309.7739, 93.098)
  line L149 (-309.7739, 93.098) -> (-309.7837, 93.0648)
  spline S107 degree 2 poles (-309.7837, 93.0648) (-309.8728, 92.9726) (-310.09, 92.6038) (-310.1573, 92.3762) knots 0 0 0 1 2 2 2
  spline S108 degree 2 poles (-310.1573, 92.3762) (-310.373, 91.6462) (-309.6518, 90.4588) (-308.7099, 90.0877) knots 0 0 0 1 2 2 2
  spline S109 degree 2 poles (-308.7099, 90.0877) (-308.8216, 90.4248) (-308.8612, 91.0757) (-308.7575, 91.4265) knots 0 0 0 1 2 2 2
  spline S110 degree 2 poles (-308.7575, 91.4265) (-308.6567, 91.7678) (-308.3679, 92.2392) (-308.0766, 92.4572) knots 0 0 0 1 2 2 2
  spline S111 degree 2 poles (-308.0766, 92.4572) (-307.7396, 92.7081) (-306.8981, 92.7996) (-306.3956, 92.6511) knots 0 0 0 1 2 2 2
  spline S112 degree 2 poles (-306.5978, 91.8449) (-306.9581, 91.9514) (-307.5024, 91.9061) (-307.7347, 91.7479) knots 0 0 0 1 2 2 2
  spline S113 degree 2 poles (-307.7347, 91.7479) (-307.9042, 91.6279) (-308.0997, 91.263) (-308.1599, 91.0591) knots 0 0 0 1 2 2 2
  spline S114 degree 2 poles (-308.1599, 91.0591) (-308.2412, 90.7842) (-308.228, 90.2184) (-308.1458, 89.9209) knots 0 0 0 1 2 2 2
  spline S115 degree 2 poles (-308.1458, 89.9209) (-308.0619, 89.891) (-307.9035, 89.8339) (-307.7802, 89.7974) knots 0 0 0 1 2 2 2
  spline S116 degree 2 poles (-307.7802, 89.7974) (-307.1734, 89.6181) (-306.3591, 89.6352) (-306.1115, 89.7579) knots 0 0 0 1 2 2 2
  spline S117 degree 2 poles (-306.1115, 89.7579) (-305.8776, 89.8691) (-305.6242, 90.186) (-305.5639, 90.3898) knots 0 0 0 1 2 2 2
  spline S118 degree 2 poles (-305.5639, 90.3898) (-305.4238, 90.8639) (-305.9246, 91.6459) (-306.5978, 91.8449) knots 0 0 0 1 2 2 2
  line L150 (-303.1707, 96.3728) -> (-304.2887, 92.781)
  line L151 (-304.2887, 92.781) -> (-305.1147, 93.0381)
  spline S119 degree 2 poles (-305.1147, 93.0381) (-305.3577, 93.5382) (-305.8181, 94.4374) (-306.0787, 94.8809) knots 0 0 0 1 2 2 2
  spline S120 degree 2 poles (-306.0787, 94.8809) (-306.6032, 95.7741) (-307.3297, 96.5335) (-307.797, 96.679) knots 0 0 0 1 2 2 2
  spline S121 degree 2 poles (-307.797, 96.679) (-308.0425, 96.7554) (-308.4576, 96.7189) (-308.6182, 96.6188) knots 0 0 0 1 2 2 2
  spline S122 degree 2 poles (-308.6182, 96.6188) (-308.7788, 96.5186) (-309.0085, 96.1966) (-309.0761, 95.9795) knots 0 0 0 1 2 2 2
  spline S123 degree 2 poles (-309.0761, 95.9795) (-309.1407, 95.7719) (-309.1691, 95.3147) (-309.1491, 95.0962) knots 0 0 0 1 2 2 2
  spline S124 degree 2 poles (-309.1491, 95.0962) (-309.1344, 94.9105) (-309.0411, 94.5449) (-309.0044, 94.43) knots 0 0 0 1 2 2 2
  line L152 (-309.0044, 94.43) -> (-309.0176, 94.3875)
  line L153 (-309.0176, 94.3875) -> (-309.8483, 94.646)
  spline S125 degree 2 poles (-309.8483, 94.646) (-309.8914, 94.9235) (-309.8538, 95.8592) (-309.7334, 96.2463) knots 0 0 0 1 2 2 2
  spline S126 degree 2 poles (-309.7334, 96.2463) (-309.4792, 97.0628) (-308.329, 97.7143) (-307.5927, 97.4852) knots 0 0 0 1 2 2 2
  spline S127 degree 2 poles (-307.5927, 97.4852) (-307.2481, 97.3779) (-306.7223, 97.0382) (-306.5209, 96.8202) knots 0 0 0 1 2 2 2
  spline S128 degree 2 poles (-306.5209, 96.8202) (-306.3101, 96.5993) (-305.9376, 96.0329) (-305.7674, 95.7314) knots 0 0 0 1 2 2 2
  spline S129 degree 2 poles (-305.7674, 95.7314) (-305.4808, 95.2384) (-304.9024, 94.0695) (-304.7359, 93.7226) knots 0 0 0 1 2 2 2
  line L154 (-304.7359, 93.7226) -> (-303.8457, 96.5829)
  line L155 (-303.8457, 96.5829) -> (-303.1707, 96.3728)
  line L156 (-301.8479, 100.4338) -> (-302.7731, 97.6054)
  line L157 (-302.7731, 97.6054) -> (-303.3651, 97.799)
  line L158 (-303.3651, 97.799) -> (-303.0209, 98.8515)
  line L159 (-303.0209, 98.8515) -> (-306.9064, 100.1225)
  line L160 (-306.9064, 100.1225) -> (-307.2506, 99.07)
  line L161 (-307.2506, 99.07) -> (-307.7815, 99.2437)
  spline S130 degree 2 poles (-307.7815, 99.2437) (-307.5863, 99.8404) (-307.7402, 100.5148) (-308.1977, 100.7061) knots 0 0 0 1 2 2 2
  line L162 (-308.1977, 100.7061) -> (-308.001, 101.3075)
  line L163 (-308.001, 101.3075) -> (-302.7765, 99.5985)
  line L164 (-302.7765, 99.5985) -> (-302.4399, 100.6274)
  line L165 (-302.4399, 100.6274) -> (-301.8479, 100.4338)
  spline S131 degree 2 poles (-302.1119, 105.787) (-301.6677, 105.6346) (-301.016, 105.0817) (-300.8485, 104.7473) knots 0 0 0 1 2 2 2
  spline S132 degree 2 poles (-300.8485, 104.7473) (-300.6703, 104.3987) (-300.6158, 103.6588) (-300.749, 103.2707) knots 0 0 0 1 2 2 2
  spline S133 degree 2 poles (-300.749, 103.2707) (-300.8821, 102.8826) (-301.3637, 102.3319) (-301.709, 102.1786) knots 0 0 0 1 2 2 2
  spline S134 degree 2 poles (-301.709, 102.1786) (-302.125, 101.9868) (-303.2925, 102.0112) (-304.0593, 102.2743) knots 0 0 0 1 2 2 2
  spline S135 degree 2 poles (-304.0593, 102.2743) (-304.8121, 102.5326) (-305.9172, 103.2567) (-306.2554, 103.7333) knots 0 0 0 1 2 2 2
  spline S136 degree 2 poles (-306.2554, 103.7333) (-306.5874, 104.1974) (-306.7382, 105.3571) (-306.5152, 106.007) knots 0 0 0 1 2 2 2
  spline S137 degree 2 poles (-306.5152, 106.007) (-306.4495, 106.1987) (-306.2966, 106.5225) (-306.2112, 106.6343) knots 0 0 0 1 2 2 2
  line L166 (-306.2112, 106.6343) -> (-305.4677, 106.3793)
  line L167 (-305.4677, 106.3793) -> (-305.479, 106.3465)
  spline S138 degree 2 poles (-305.479, 106.3465) (-305.572, 106.2582) (-305.8049, 105.8992) (-305.8819, 105.6747) knots 0 0 0 1 2 2 2
  spline S139 degree 2 poles (-305.8819, 105.6747) (-306.129, 104.9547) (-305.4597, 103.7373) (-304.5347, 103.3258) knots 0 0 0 1 2 2 2
  spline S140 degree 2 poles (-304.5347, 103.3258) (-304.6317, 103.6675) (-304.6432, 104.3195) (-304.5245, 104.6655) knots 0 0 0 1 2 2 2
  spline S141 degree 2 poles (-304.5245, 104.6655) (-304.409, 105.0021) (-304.1001, 105.4606) (-303.7997, 105.6658) knots 0 0 0 1 2 2 2
  spline S142 degree 2 poles (-303.7997, 105.6658) (-303.4522, 105.902) (-302.6075, 105.9571) (-302.1119, 105.787) knots 0 0 0 1 2 2 2
  spline S143 degree 2 poles (-302.3487, 104.9903) (-302.7041, 105.1122) (-303.2498, 105.0904) (-303.4887, 104.9424) knots 0 0 0 1 2 2 2
  spline S144 degree 2 poles (-303.4887, 104.9424) (-303.6633, 104.8299) (-303.8743, 104.4737) (-303.9433, 104.2727) knots 0 0 0 1 2 2 2
  spline S145 degree 2 poles (-303.9433, 104.2727) (-304.0363, 104.0015) (-304.0476, 103.4357) (-303.9783, 103.1349) knots 0 0 0 1 2 2 2
  spline S146 degree 2 poles (-303.9783, 103.1349) (-303.8957, 103.1014) (-303.74, 103.0375) (-303.6184, 102.9958) knots 0 0 0 1 2 2 2
  spline S147 degree 2 poles (-303.6184, 102.9958) (-303.0199, 102.7904) (-302.2056, 102.7723) (-301.9529, 102.8842) knots 0 0 0 1 2 2 2
  spline S148 degree 2 poles (-301.9529, 102.8842) (-301.7144, 102.9853) (-301.4476, 103.2909) (-301.3786, 103.492) knots 0 0 0 1 2 2 2
  spline S149 degree 2 poles (-301.3786, 103.492) (-301.2181, 103.9595) (-301.6848, 104.7625) (-302.3487, 104.9903) knots 0 0 0 1 2 2 2
  spline S150 degree 2 poles (-295.2983, 126.2884) (-294.5275, 125.966) (-293.5483, 124.8225) (-293.4211, 124.1531) knots 0 0 0 1 2 2 2
  spline S151 degree 2 poles (-293.4211, 124.1531) (-293.3313, 123.6119) (-293.5169, 122.6554) (-293.803, 121.9713) knots 0 0 0 1 2 2 2
  line L168 (-293.803, 121.9713) -> (-294.3446, 120.6761)
  line L169 (-294.3446, 120.6761) -> (-299.9724, 123.0295)
  line L170 (-299.9724, 123.0295) -> (-299.4364, 124.3111)
  spline S152 degree 2 poles (-299.4364, 124.3111) (-299.1046, 125.1046) (-298.4898, 125.9084) (-298.1466, 126.1399) knots 0 0 0 1 2 2 2
  spline S153 degree 2 poles (-298.1466, 126.1399) (-297.5593, 126.532) (-296.1192, 126.6316) (-295.2983, 126.2884) knots 0 0 0 1 2 2 2
  spline S154 degree 2 poles (-295.6335, 125.5123) (-296.2811, 125.7831) (-297.3771, 125.7378) (-297.8144, 125.4223) knots 0 0 0 1 2 2 2
  spline S155 degree 2 poles (-297.8144, 125.4223) (-298.1181, 125.1957) (-298.5619, 124.583) (-298.7736, 124.0767) knots 0 0 0 1 2 2 2
  line L171 (-298.7736, 124.0767) -> (-299.012, 123.5067)
  line L172 (-299.012, 123.5067) -> (-294.6795, 121.6949)
  line L173 (-294.6795, 121.6949) -> (-294.4411, 122.2649)
  spline S156 degree 2 poles (-294.4411, 122.2649) (-294.2332, 122.762) (-294.0781, 123.5813) (-294.1647, 123.9765) knots 0 0 0 1 2 2 2
  spline S157 degree 2 poles (-294.1647, 123.9765) (-294.2652, 124.4793) (-294.9768, 125.2377) (-295.6335, 125.5123) knots 0 0 0 1 2 2 2
  line L174 (-291.2863, 127.868) -> (-292.228, 125.7009)
  line L175 (-292.228, 125.7009) -> (-292.7993, 125.9491)
  line L176 (-292.7993, 125.9491) -> (-292.49, 126.6609)
  line L177 (-292.49, 126.6609) -> (-296.942, 128.5956)
  line L178 (-296.942, 128.5956) -> (-297.2514, 127.8838)
  line L179 (-297.2514, 127.8838) -> (-297.8226, 128.1321)
  line L180 (-297.8226, 128.1321) -> (-296.8809, 130.2992)
  line L181 (-296.8809, 130.2992) -> (-296.3096, 130.0509)
  line L182 (-296.3096, 130.0509) -> (-296.6189, 129.3391)
  line L183 (-296.6189, 129.3391) -> (-292.1668, 127.4044)
  line L184 (-292.1668, 127.4044) -> (-291.8575, 128.1162)
  line L185 (-291.8575, 128.1162) -> (-291.2863, 127.868)
  line L186 (-288.7328, 133.5543) -> (-289.0671, 132.8157)
  line L187 (-289.0671, 132.8157) -> (-293.8543, 134.9824)
  line L188 (-293.8543, 134.9824) -> (-291.2546, 132.0586)
  line L189 (-291.2546, 132.0586) -> (-291.4584, 131.6083)
  line L190 (-291.4584, 131.6083) -> (-295.3647, 131.6454)
  line L191 (-295.3647, 131.6454) -> (-290.5775, 129.4786)
  line L192 (-290.5775, 129.4786) -> (-290.8893, 128.7896)
  line L193 (-290.8893, 128.7896) -> (-296.4466, 131.3049)
  line L194 (-296.4466, 131.3049) -> (-295.99, 132.3137)
  line L195 (-295.99, 132.3137) -> (-292.2683, 132.3004)
  line L196 (-292.2683, 132.3004) -> (-294.7548, 135.0428)
  line L197 (-294.7548, 135.0428) -> (-294.2901, 136.0695)
  line L198 (-294.2901, 136.0695) -> (-288.7328, 133.5543)
  line L199 (-287.2978, 136.594) -> (-288.3044, 134.4562)
  line L200 (-288.3044, 134.4562) -> (-288.8679, 134.7216)
  line L201 (-288.8679, 134.7216) -> (-288.5373, 135.4237)
  line L202 (-288.5373, 135.4237) -> (-292.929, 137.4918)
  line L203 (-292.929, 137.4918) -> (-293.2596, 136.7897)
  line L204 (-293.2596, 136.7897) -> (-293.8231, 137.0551)
  line L205 (-293.8231, 137.0551) -> (-292.8165, 139.1928)
  line L206 (-292.8165, 139.1928) -> (-292.253, 138.9274)
  line L207 (-292.253, 138.9274) -> (-292.5836, 138.2253)
  line L208 (-292.5836, 138.2253) -> (-288.1919, 136.1572)
  line L209 (-288.1919, 136.1572) -> (-287.8613, 136.8593)
  line L210 (-287.8613, 136.8593) -> (-287.2978, 136.594)
  line L211 (-286.2455, 138.7811) -> (-291.082, 141.1337)
  line L212 (-291.082, 141.1337) -> (-291.9772, 139.2933)
  line L213 (-291.9772, 139.2933) -> (-292.6262, 139.609)
  line L214 (-292.6262, 139.609) -> (-290.4812, 144.0187)
  line L215 (-290.4812, 144.0187) -> (-289.8322, 143.7031)
  line L216 (-289.8322, 143.7031) -> (-290.7274, 141.8627)
  line L217 (-290.7274, 141.8627) -> (-285.8909, 139.5101)
  line L218 (-285.8909, 139.5101) -> (-286.2455, 138.7811)
  line L219 (-282.5834, 146.1186) -> (-283.0589, 145.1792)
  line L220 (-283.0589, 145.1792) -> (-286.0951, 144.5554)
  line L221 (-286.0951, 144.5554) -> (-286.5149, 143.7263)
  line L222 (-286.5149, 143.7263) -> (-284.3494, 142.63)
  line L223 (-284.3494, 142.63) -> (-284.7155, 141.9067)
  line L224 (-284.7155, 141.9067) -> (-290.1579, 144.6618)
  line L225 (-290.1579, 144.6618) -> (-289.4479, 146.0643)
  spline S158 degree 2 poles (-289.4479, 146.0643) (-289.2113, 146.5318) (-288.7906, 147.1112) (-288.4602, 147.3041) knots 0 0 0 1 2 2 2
  spline S159 degree 2 poles (-288.4602, 147.3041) (-288.1299, 147.497) (-287.3846, 147.5353) (-286.9568, 147.3187) knots 0 0 0 1 2 2 2
  spline S160 degree 2 poles (-286.9568, 147.3187) (-286.3614, 147.0173) (-285.8625, 146.0001) (-285.9319, 145.3814) knots 0 0 0 1 2 2 2
  line L226 (-285.9319, 145.3814) -> (-282.5834, 146.1186)
  spline S161 degree 2 poles (-287.2813, 146.5355) (-287.5195, 146.6561) (-287.9704, 146.6738) (-288.1787, 146.5576) knots 0 0 0 1 2 2 2
  spline S162 degree 2 poles (-288.1787, 146.5576) (-288.3583, 146.4546) (-288.6498, 146.0869) (-288.8016, 145.787) knots 0 0 0 1 2 2 2
  line L227 (-288.8016, 145.787) -> (-289.1655, 145.0681)
  line L228 (-289.1655, 145.0681) -> (-287.1191, 144.0321)
  line L229 (-287.1191, 144.0321) -> (-286.7976, 144.6672)
  spline S163 degree 2 poles (-286.7976, 144.6672) (-286.6391, 144.9804) (-286.497, 145.5346) (-286.582, 145.7936) knots 0 0 0 1 2 2 2
  spline S164 degree 2 poles (-286.582, 145.7936) (-286.6515, 146.0283) (-286.999, 146.3926) (-287.2813, 146.5355) knots 0 0 0 1 2 2 2
  line L230 (-281.3665, 148.4277) -> (-282.4613, 146.3338)
  line L231 (-282.4613, 146.3338) -> (-283.0132, 146.6223)
  line L232 (-283.0132, 146.6223) -> (-282.6537, 147.3101)
  line L233 (-282.6537, 147.3101) -> (-286.9555, 149.5591)
  line L234 (-286.9555, 149.5591) -> (-287.3151, 148.8713)
  line L235 (-287.3151, 148.8713) -> (-287.8671, 149.1599)
  line L236 (-287.8671, 149.1599) -> (-286.7723, 151.2539)
  line L237 (-286.7723, 151.2539) -> (-286.2204, 150.9653)
  line L238 (-286.2204, 150.9653) -> (-286.5799, 150.2775)
  line L239 (-286.5799, 150.2775) -> (-282.2781, 148.0285)
  line L240 (-282.2781, 148.0285) -> (-281.9185, 148.7163)
  line L241 (-281.9185, 148.7163) -> (-281.3665, 148.4277)
  spline S165 degree 2 poles (-279.9971, 150.7613) (-280.3111, 150.1781) (-280.9955, 149.4911) (-281.3641, 149.2236) knots 0 0 0 1 2 2 2
  line L242 (-281.3641, 149.2236) -> (-282.2607, 149.7065)
  line L243 (-282.2607, 149.7065) -> (-282.2326, 149.7587)
  spline S166 degree 2 poles (-282.2326, 149.7587) (-281.712, 149.9331) (-280.8659, 150.6284) (-280.6432, 151.0419) knots 0 0 0 1 2 2 2
  spline S167 degree 2 poles (-280.6432, 151.0419) (-280.3245, 151.6338) (-280.4905, 152.5036) (-280.8953, 152.7216) knots 0 0 0 1 2 2 2
  spline S168 degree 2 poles (-280.8953, 152.7216) (-281.2174, 152.8951) (-281.7889, 152.793) (-282.0741, 152.503) knots 0 0 0 1 2 2 2
  spline S169 degree 2 poles (-282.0741, 152.503) (-282.2774, 152.2925) (-282.5958, 151.9305) (-282.8405, 151.6637) knots 0 0 0 1 2 2 2
  spline S170 degree 2 poles (-282.8405, 151.6637) (-283.0645, 151.425) (-283.5232, 151.105) (-283.793, 151.0313) knots 0 0 0 1 2 2 2
  spline S171 degree 2 poles (-283.793, 151.0313) (-284.0606, 150.962) (-284.6377, 151.037) (-284.9511, 151.2058) knots 0 0 0 1 2 2 2
  spline S172 degree 2 poles (-284.9511, 151.2058) (-285.604, 151.5574) (-285.939, 153.0516) (-285.5148, 153.8394) knots 0 0 0 1 2 2 2
  spline S173 degree 2 poles (-285.5148, 153.8394) (-285.2711, 154.292) (-284.6614, 154.9967) (-284.3065, 155.2492) knots 0 0 0 1 2 2 2
  line L244 (-284.3065, 155.2492) -> (-283.4534, 154.7898)
  line L245 (-283.4534, 154.7898) -> (-283.4815, 154.7375)
  spline S174 degree 2 poles (-283.4815, 154.7375) (-283.8549, 154.6073) (-284.6343, 153.994) (-284.871, 153.5544) knots 0 0 0 1 2 2 2
  spline S175 degree 2 poles (-284.871, 153.5544) (-285.1382, 153.0582) (-285.003, 152.1938) (-284.6243, 151.9899) knots 0 0 0 1 2 2 2
  spline S176 degree 2 poles (-284.6243, 151.9899) (-284.2848, 151.8071) (-283.6855, 151.9503) (-283.4113, 152.2406) knots 0 0 0 1 2 2 2
  spline S177 degree 2 poles (-283.4113, 152.2406) (-283.2285, 152.4341) (-282.7179, 153.0069) (-282.5355, 153.1894) knots 0 0 0 1 2 2 2
  spline S178 degree 2 poles (-282.5355, 153.1894) (-282.0681, 153.6507) (-281.1082, 153.7963) (-280.6077, 153.5268) knots 0 0 0 1 2 2 2
  spline S179 degree 2 poles (-280.6077, 153.5268) (-280.2899, 153.3557) (-279.8189, 152.7708) (-279.7299, 152.4253) knots 0 0 0 1 2 2 2
  spline S180 degree 2 poles (-279.7299, 152.4253) (-279.6331, 152.0419) (-279.7322, 151.2531) (-279.9971, 150.7613) knots 0 0 0 1 2 2 2
  line L246 (-275.2037, 159.5813) -> (-275.7244, 158.6662)
  line L247 (-275.7244, 158.6662) -> (-279.2931, 158.1317)
  line L248 (-279.2931, 158.1317) -> (-279.1211, 157.6244)
  line L249 (-279.1211, 157.6244) -> (-277.003, 156.4191)
  line L250 (-277.003, 156.4191) -> (-277.4039, 155.7145)
  line L251 (-277.4039, 155.7145) -> (-282.7057, 158.7312)
  line L252 (-282.7057, 158.7312) -> (-282.3048, 159.4359)
  line L253 (-282.3048, 159.4359) -> (-279.8687, 158.0497)
  line L254 (-279.8687, 158.0497) -> (-281.0678, 161.6099)
  line L255 (-281.0678, 161.6099) -> (-280.5789, 162.4692)
  line L256 (-280.5789, 162.4692) -> (-279.4608, 158.9267)
  line L257 (-279.4608, 158.9267) -> (-275.2037, 159.5813)
  line L258 (-275.2904, 159.4316) -> (-279.4989, 164.3027)
  line L259 (-279.4989, 164.3027) -> (-278.9914, 165.1627)
  line L260 (-278.9914, 165.1627) -> (-272.6928, 163.8337)
  line L261 (-272.6928, 163.8337) -> (-273.1274, 163.0972)